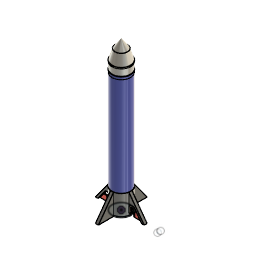
Zephyr I v11 (Autodesk Fusion 360 design; units mm, degrees)
Autodesk Fusion 360 part; units mm, degrees
note: some values were not read from the file. Chosen so that the rebuilt part matches the saved one: which bodies a step acts on; which face or edge a step refers to.
sketch "Szkic1" plane through (0, 0, 0) normal (0, 0, 1) x (1, 0, 0)
  circle A0 centre (0, 0) radius 9
  circle A1 centre (0, 0) radius 37.5
  dimension "d1" = 18
  dimension "d2" = 75
  constraint coincident A0.centre A1.centre
  constraint concentric A0 A1
  measures "d1" diameter of A0
  measures "d2" diameter of A1
extrude "Wyciągnięcie proste1" add sketch "Szkic1" along normal blind 99 makes body 1
sketch "Szkic2" plane through (0, 0, 0) normal (0, 0, 1) x (1, 0, 0)
  circle A0 centre (0, 0) radius 9
  dimension "d5" = 18
  constraint coincident A0.centre origin
  measures "d5" diameter of A0
extrude "Wyciągnięcie proste2" add sketch "Szkic2" along normal blind 30 bodies 1
move_body "Przesuń1" bodies 1 to x (-1, 0, 0) y (0, 1, 0) z (0, 0, -1) at (0, 0, 100)
sketch "Szkic3" plane through (0, 0, 0) normal (0, 1, 0) x (1, 0, 0)
move_face "Odsuń powierzchnie1" offset -20 1 faces at (-8.8919, -13.3334, 100) on bodies 1
sketch "Szkic4" plane through (0, 0, 0) normal (0, 1, 0) x (1, 0, 0)
  line L0 (0, 0) -> (6.25, 0)
  line L1 (0, 0) -> (-6.25, 0)
  line L2 (6.25, 0) -> (6.25, -22.4)
  line L3 (-6.25, 0) -> (-6.25, -22.4)
  line L4 (-6.25, -22.4) -> (6.25, -22.4)
  dimension "d9" = 6.25
  dimension "d10" = 6.25
  dimension "d11" = 22.4
  dimension "d12" = 22.4
  constraint coincident L0.start L1.start
  constraint horizontal L0
  constraint parallel L0 L1
  constraint perpendicular L0 L2
  constraint perpendicular L1 L3
  measures "d9" distance of L0.start L0.end
  measures "d10" distance of L0.start L1.end
  measures "d11" distance of L0.end L2.end
  measures "d12" distance of L1.end L3.end
move_body "Przesuń2" bodies 1 to x (1, 0, 0) y (0, 1, 0) z (0, 0, 1) at (0, 0, -10)
move_body "Przesuń3" bodies 1 to x (1, 0, 0) y (0, 1, 0) z (0, 0, 1) at (0, -40, 0)
move_body "Przesuń4" bodies 1 to x (1, 0, 0) y (0, 1, 0) z (0, 0, 1) at (0, 2.5, 0)
extrude "Wyciągnięcie proste3" cut sketch "Szkic4" against normal blind 19.8 bodies 1
move_body "Przesuń5" bodies 1 to x (1, 0, 0) y (0, 1, 0) z (0, 0, 1) at (0, -2.5, 0)
move_body "Przesuń6" bodies 1 to x (1, 0, 0) y (0, 1, 0) z (0, 0, 1) at (0, 40, 0)
sketch "Szkic6" plane through (0, 0, 0) normal (1, 0, 0) x (0, 1, 0)
  line L0 (0, 0) -> (-6.25, 0)
  line L1 (0, 0) -> (6.25, 0)
  line L2 (6.25, 0) -> (6.25, 22.4)
  line L3 (-6.25, 0) -> (-8, 0)
  line L4 (-8, 0) -> (-8, 22.4)
  line L5 (-8, 22.4) -> (-6.25, 22.4)
  line L6 (-6.25, 22.4) -> (-6.25, 0)
  line L7 (-6.25, 22.4) -> (6.25, 22.4)
  dimension "d22" = 6.25
  dimension "d23" = 6.25
  dimension "d24" = 22.4
  dimension "d25" = 22.4
  constraint coincident L0.start L1.start
  constraint horizontal L0
  constraint parallel L0 L1
  constraint perpendicular L1 L2
  constraint horizontal L3
  constraint vertical L4
  constraint horizontal L5
  constraint vertical L6
  measures "d22" distance of L0.start L0.end
  measures "d23" distance of L0.start L1.end
  measures "d24" distance of L1.end L2.end
  measures "d25" distance of L0.end L5.end
move_body "Przesuń10" bodies 1 to x (0, 1, 0) y (-1, 0, 0) z (0, 0, 1) at (0, 0, 0)
move_body "Przesuń11" bodies 1 to x (1, 0, 0) y (0, 1, 0) z (0, 0, 1) at (-40, 0, 0)
move_body "Przesuń12" bodies 1 to x (1, 0, 0) y (0, 1, 0) z (0, 0, 1) at (2.5, 0, 0)
extrude "Wyciągnięcie proste5" cut sketch "Szkic6" against normal blind 19.8 contours L0 L1 L2 L6 L7 bodies 1
move_body "Przesuń13" bodies 1 to x (1, 0, 0) y (0, 1, 0) z (0, 0, 1) at (2.5, 0, 0)
move_body "Przesuń14" bodies 1 to x (1, 0, 0) y (0, 1, 0) z (0, 0, 1) at (-2.5, 0, 0)
move_body "Przesuń15" bodies 1 to x (1, 0, 0) y (0, 1, 0) z (0, 0, 1) at (-2.5, 0, 0)
move_body "Przesuń16" bodies 1 to x (1, 0, 0) y (0, 1, 0) z (0, 0, 1) at (40, 0, 0)
sketch "Szkic7" plane through (0, 0, 0) normal (1, 0, 0) x (0, 1, 0)
  line L0 (-6.25, 0, 150) -> (6.25, 0, 150)
sketch "Szkic8" plane through (0, 0, 0) normal (0, 0, 1) x (1, 0, 0)
  line L0 (17.7, 6.25) -> (17.7, -6.25)
  line L1 (17.7, -6.25) -> (22.7, -6.25)
  line L2 (22.7, -6.25) -> (22.7, 6.25)
  line L3 (17.7, 6.25) -> (22.7, 6.25)
  line L4 (-17.7, 6.25) -> (-17.7, -6.25)
  line L5 (-17.7, -6.25) -> (-22.7, -6.25)
  line L6 (-22.7, -6.25) -> (-22.7, 6.25)
  line L7 (-22.7, 6.25) -> (-17.7, 6.25)
  dimension "d28" = 12.5
  dimension "d29" = 5
  dimension "d30" = 12.5
  dimension "d31" = 12.5
  dimension "d32" = 5
  dimension "d33" = 12.5
  constraint vertical L0
  constraint perpendicular L0 L1
  constraint perpendicular L1 L2
  constraint vertical L4
  constraint perpendicular L4 L5
  constraint perpendicular L5 L6
  measures "d28" distance of L0.start L0.end
  measures "d29" distance of L0.end L1.end
  measures "d30" distance of L1.end L2.end
  measures "d31" distance of L4.start L4.end
  measures "d32" distance of L4.end L5.end
  measures "d33" distance of L5.end L6.end
extrude "Wyciągnięcie proste6" cut sketch "Szkic8" along normal blind 90 bodies 1
other "Element bazowy siatki1"
other "Element bazowy siatki2"
other "Element bazowy siatki3"
other "Zmień1"
other "Zmień2"
other "Kopiowanie i wklejenie siatek1"
other "Zmień3"
other "Zmień4"
other "Zmień5"
other "Zmień6"
other "Zmień7"
other "Zmień8"
other "Zmień9"
other "Kopiowanie i wklejenie siatek2"
other "Zmień10"
other "Zmień11"
other "Zmień12"
other "Zmień13"
other "Zmień14"
other "Zmień15"
move_body "Przesuń17" bodies 1 to x (1, 0, 0) y (0, 1, 0) z (0, 0, 1) at (0, 0, 10)
other "Zmień16"
sketch "Szkic9" plane through (0, 0, 0) normal (0, 1, 0) x (1, 0, 0)
  line L0 (37.5, -80) -> (95.7821, 0.0262)
  line L1 (-37.5, -80) -> (-95.8898, -0.0523)
  line L2 (-95.8898, -0.0523) -> (-85.8898, -0.0523)
  line L3 (95.7821, 0.0262) -> (85.7821, 0.0262)
  line L4 (37.5, -80) -> (37.5, -37.25)
  line L5 (37.5, -37.25) -> (68.6343, -37.25)
  line L6 (-37.5, -37.2753) -> (-37.5, -80)
  line L7 (-37.5, -37.2753) -> (-68.704, -37.2753)
  line L8 (37.5, -37.25) -> (-37.5, -37.2753)
  line L9 (-37.5, -37.25) -> (-68.7225, -37.25)
  line L10 (85.7821, 0.0262) -> (58.6343, -37.25)
  line L11 (-85.8898, -0.0523) -> (-58.7225, -37.25)
  dimension "d36" = 99
  dimension "d37" = 99
  dimension "d38" = 10
  dimension "d39" = 10
  constraint horizontal L2
  constraint horizontal L3
  constraint vertical L4
  constraint coincident L0 L5.end
  constraint perpendicular L4 L5
  constraint perpendicular L5 L6
  constraint coincident L1 L7.end
  constraint perpendicular L6 L7
  constraint coincident L1 L9.end
  constraint perpendicular L6 L9
  constraint coincident L5 L10.end
  constraint parallel L0 L10
  constraint coincident L9 L11.end
  constraint parallel L1 L11
  measures "d36" distance of L0.start L0.end
  measures "d37" distance of L1.start L1.end
  measures "d38" distance of L1.end L2.end
  measures "d39" distance of L0.end L3.end
move_body "Przesuń18" bodies 1 to x (1, 0, 0) y (0, 1, 0) z (0, 0, 1) at (0, -50, 0)
extrude "Wyciągnięcie proste7" add sketch "Szkic9" along normal blind 6 separate body makes body 2 at (-47.9013, 0, 51.5169) makes body 3 at (-83.5007, 0, 12.4515) makes body 4 at (44.5448, 6, 51.5)
extrude "Wyciągnięcie proste8" add 3 faces at (-83.5007, 0, 12.4515) (-47.9013, 0, 51.5169) (44.5448, 0, 51.5) along direction (0, -1, 0) blind 6 on bodies 2 3 4 bodies 3 2 4
combine "Kombinacja1" operation add target body 2 tool bodies 3 makes body 5 at (-86.834, 2, 12.4515)
move_body "Przesuń19" bodies 1 to x (1, 0, 0) y (0, 1, 0) z (0, 0, 1) at (0, 50, 0)
combine "Kombinacja2" operation add target body 5 tool bodies 2 makes body 6 at (-47.9013, 6, 51.5169)
move_face "Odsuń powierzchnie2" offset 0.028 1 faces at (-58.3027, 2, 37.2753) on bodies 6
combine "Kombinacja3" operation add target body 6 tool bodies 5
copy_body "Kopiuj-wklej bryły2" bodies 4 6 makes body 7 makes body 8
move_body "Przesuń21" bodies 7 8 to x (1, 0, 0) y (0, 1, 0) z (0, 0, 1) at (0, 0, 0)
copy_body "Kopiuj-wklej bryły3" bodies 1 makes body 9
move_body "Przesuń22" bodies 9 to x (1, 0, 0) y (0, 1, 0) z (0, 0, 1) at (0, 0, 0)
sketch "Szkic10" plane through (0, 0, 0) normal (0, 0, 1) x (1, 0, 0)
  circle A0 centre (0, 0) radius 37.5
  dimension "d47" = 75
  constraint coincident A0.centre origin
  measures "d47" diameter of A0
extrude "Wyciągnięcie proste9" add sketch "Szkic10" along normal blind 1 separate body makes body 10
move_body "Przesuń23" bodies 10 7 6 to x (0, -1, 0) y (1, 0, 0) z (0, 0, 1) at (0, 0, 0)
combine "Kombinacja4" operation add target body 10 tool bodies 9
combine "Kombinacja5" operation add target body 1 tool bodies 10
move_face "Odsuń powierzchnie5" offset 37.2 2 faces at (-2, 44.5748, 37.2473) (2, -51.5895, 37.25) on bodies 6 7
sketch "Szkic11" plane through (0, 0, 0) normal (0, 0, 1) x (1, 0, 0)
  circle A0 centre (0, 0) radius 9
  dimension "d51" = 18
  constraint coincident A0.centre origin
  measures "d51" diameter of A0
extrude "Wyciągnięcie proste10" cut sketch "Szkic11" along normal blind 10 bodies 1
sketch "Szkic12" plane through (0, 0, 0) normal (0, 0, 1) x (1, 0, 0)
  circle A0 centre (0, 0) radius 37.5
  dimension "d54" = 75
  constraint coincident A0.centre origin
  measures "d54" diameter of A0
combine "Kombinacja6" operation add target body 4 tool bodies 1
combine "Kombinacja7" operation add target body 4 tool bodies 6
combine "Kombinacja8" operation add target body 4 tool bodies 8
combine "Kombinacja9" operation add target body 7 tool bodies 4
move_body "Przesuń24" bodies 7 to x (1, 0, 0) y (0, 1, 0) z (0, 0, 1) at (0, 0, -80)
other "Zmień17"
sketch "Szkic13" plane through (0, 0, 0) normal (0, 0, 1) x (1, 0, 0)
  circle A0 centre (0, 0) radius 36.5
  dimension "d55" = 73
  constraint coincident A0.centre origin
  measures "d55" diameter of A0
extrude "Wyciągnięcie proste11" add sketch "Szkic12" along normal blind 400 separate body makes body 11
sketch "Szkic14" plane through (0, 0, 0) normal (0, 0, 1) x (1, 0, 0)
  circle A0 centre (0, 0) radius 36.5
  dimension "d58" = 73
  constraint coincident A0.centre origin
  measures "d58" diameter of A0
extrude "Wyciągnięcie proste12" cut sketch "Szkic13" along normal blind 500 bodies 11
sketch "Szkic15" plane through (0, 0, 0) normal (0, 0, 1) x (1, 0, 0)
  circle A0 centre (0, 0) radius 10
  circle A1 centre (0, 0) radius 9
  dimension "d61" = 20
  dimension "d62" = 18
  constraint coincident A0.centre A1.centre
  constraint concentric A0 A1
  measures "d61" diameter of A0
  measures "d62" diameter of A1
extrude "Wyciągnięcie proste13" cut sketch "Szkic15" against normal blind 130 bodies 7 makes body 12 at (6, -53.5755, -53.3) makes body 12 at (-36.0833, 10.2102, -42.5333) makes body 12 at (-76.4265, 0.0026, -53.2985) makes body 12 at (-6, 56.9645, -53.3018) makes body 12 at (76.3547, -0.0026, -53.3508)
sketch "Szkic16" plane through (0, 0, 0) normal (0, 0, 1) x (1, 0, 0)
  circle A0 centre (0, 0) radius 10
  circle A1 centre (0, 0) radius 9
  dimension "d65" = 20
  dimension "d66" = 18
  constraint coincident A0.centre A1.centre
  constraint concentric A0 A1
  measures "d65" diameter of A0
  measures "d66" diameter of A1
move_body "Przesuń25" bodies 12 11 to x (1, 0, 0) y (0, 1, 0) z (0, 0, 1) at (0, -120, 0)
other "Zmień18"
extrude "Wyciągnięcie proste14" add sketch "Szkic16" against normal blind 80 bodies 7
move_body "Przesuń26" bodies 11 12 to x (1, 0, 0) y (0, 1, 0) z (0, 0, 1) at (0, 120, 0)
other "Zmień19"
move_body "Przesuń27" bodies 11 12 to x (1, 0, 0) y (0, 1, 0) z (0, 0, 1) at (0, 0, 80)
other "Zmień20"
move_body "Przesuń28" bodies 7 to x (1, 0, 0) y (0, 1, 0) z (0, 0, 1) at (0, 0, 80)
sketch "Szkic17" plane through (0, 0, 0) normal (0, 1, 0) x (1, 0, 0)
  line L0 (54.3, 0.55) -> (54.3, -36.5257)
  line L1 (54.3, -36.5257) -> (58.3, -36.5257)
  line L2 (58.3, -36.5257) -> (85, 0)
  line L3 (85, 0) -> (54.3, 0.55)
  line L4 (-53.9, 0.55) -> (-54.1253, -36.5257)
  line L5 (-54.1253, -36.5257) -> (-58.1253, -36.5014)
  line L6 (-58.1253, -36.5014) -> (-85, 0)
  line L7 (-85, 0) -> (-53.9, 0.55)
  line L8 (-54.0249, -19.9942) -> (-70.2789, -19.9942)
  line L9 (54.3, -19.9942) -> (70.3844, -19.9942)
  dimension "d69" = 4
  dimension "d70" = 4
  constraint vertical L0
  constraint perpendicular L0 L1
  constraint perpendicular L4 L5
  constraint coincident L4 L8.start
  constraint coincident L6 L8.end
  constraint horizontal L8
  constraint coincident L0 L9.start
  constraint coincident L2 L9.end
  constraint perpendicular L0 L9
  measures "d69" distance of L0.end L1.end
  measures "d70" distance of L4.end L5.end
extrude "Wyciągnięcie proste15" add sketch "Szkic17" along normal blind 2 separate body contours L0 L2 L3 L9 | L4 L6 L7 L8 makes body 13 at (-69.7263, 0, 6.4814) makes body 14 at (69.8948, 0, 6.4814)
move_face "Odsuń powierzchnie6" offset 2 2 faces at (-69.7263, 0, 6.4814) (69.8948, 0, 6.4814) on bodies 13 14
move_body "Przesuń29" bodies 14 11 12 13 7 to x (1, 0, 0) y (0, 1, 0) z (0, 0, 1) at (0, 0, -480)
other "Zmień21"
move_body "Przesuń30" bodies 7 14 13 12 11 to x (1, 0, 0) y (0, 1, 0) z (0, 0, 1) at (0, 0, -25)
other "Zmień22"
sketch "Szkic19" plane through (0, 0, 0) normal (0, 0, 1) x (1, 0, 0)
  circle A0 centre (0, 0) radius 36.5
  circle A1 centre (0, 0) radius 37.5
  circle A2 centre (0, 0) radius 35.5
  dimension "d75" = 73
  dimension "d76" = 75
  dimension "d77" = 71
  constraint coincident A0.centre A1.centre
  constraint concentric A0 A2
  measures "d75" diameter of A0
  measures "d76" diameter of A1
  measures "d77" diameter of A2
extrude "Wyciągnięcie proste16" add sketch "Szkic19" against normal blind 10 separate body contours A0 makes body 15
sketch "Szkic20" plane through (0, 0, 0) normal (0, 0, 1) x (1, 0, 0)
  circle A0 centre (0, 0) radius 37.5
  dimension "d80" = 75
  constraint coincident A0.centre origin
  measures "d80" diameter of A0
extrude "Wyciągnięcie proste17" add sketch "Szkic20" along normal blind 2 bodies 15
move_body "Przesuń31" bodies 15 to x (1, 0, 0) y (0, 1, 0) z (0, 0, 1) at (0, 0, -2)
sketch "Szkic21" plane through (0, 0, 0) normal (0, 0, 1) x (1, 0, 0)
  circle A0 centre (0, 0) radius 37.5
  circle A1 centre (0, 0) radius 36.5
  dimension "d83" = 75
  dimension "d84" = 73
  constraint coincident A0.centre A1.centre
  measures "d83" diameter of A0
  measures "d84" diameter of A1
extrude "Wyciągnięcie proste18" add sketch "Szkic21" along normal blind 30 bodies 15
move_body "Przesuń32" bodies 15 11 12 14 13 to x (1, 0, 0) y (0, 1, 0) z (0, 0, 1) at (0, 0, -40)
other "Zmień23"
sketch "Szkic22" plane through (0, 0, 0) normal (0, 1, 0) x (1, 0, 0)
  line L0 (0, 0) -> (37.5, 0)
  line L1 (0, 0) -> (0, -75)
  line L2 (37.5, 0) -> (25, -40)
  line L3 (25, -40) -> (0, -75)
  dimension "d87" = 37.5
  dimension "d88" = 75
  constraint coincident L0.start L1.start
  constraint horizontal L0
  constraint perpendicular L0 L1
  measures "d87" distance of L0.start L0.end
  measures "d88" distance of L0.start L1.end
revolve "Obrót1" add sketch "Szkic22" angle 360 about axis through (0, 0, 0) along (0, 0, 1) separate body makes body 16
sketch "Szkic23" plane through (0, 0, 0) normal (0, 0, 1) x (1, 0, 0)
  circle A0 centre (0, 0) radius 36.5
  dimension "d90" = 73
  constraint coincident A0.centre origin
  measures "d90" diameter of A0
sketch "Szkic24" plane through (0, 0, 0) normal (0, 0, 1) x (1, 0, 0)
  circle A0 centre (0, 0) radius 35.5
  dimension "d91" = 71
  constraint coincident A0.centre origin
  measures "d91" diameter of A0
extrude "Wyciągnięcie proste19" add sketch "Szkic14" against normal blind 5 bodies 16
move_body "Przesuń33" bodies 16 to x (1, 0, 0) y (0, 1, 0) z (0, 0, 1) at (0, 0, 50)
sketch "Szkic25" plane through (0, 0, 0) normal (0, 0, 1) x (1, 0, 0)
  circle A0 centre (0, 0) radius 35.5
  dimension "d94" = 71
  constraint coincident A0.centre origin
  measures "d94" diameter of A0
extrude "Wyciągnięcie proste20" cut sketch "Szkic25" along normal blind 50 bodies 16
move_body "Przesuń34" bodies 13 12 14 15 16 to x (1, 0, 0) y (0, 1, 0) z (0, 0, 1) at (0, 0, 545)
other "Zmień24"
move_body "Przesuń35" bodies 11 to x (1, 0, 0) y (0, 1, 0) z (0, 0, 1) at (0, 0, 550)
move_body "Przesuń36" bodies 7 to x (1, 0, 0) y (0, 1, 0) z (0, 0, 1) at (0, 0, 505)
move_body "Przesuń37" bodies 11 to x (1, 0, 0) y (0, 1, 0) z (0, 0, 1) at (0, 0, -5)
move_body "Przesuń38" bodies 15 to x (1, 0, 0) y (0, 1, 0) z (0, 0, 1) at (0, 0, -23)
move_body "Przesuń39" bodies 16 to x (1, 0, 0) y (0, 1, 0) z (0, 0, 1) at (0, 0, -83)
split "Podział1" by face at (-36.0833, 10.2102, 37.4667) of body 12 bodies 12 makes body 17 at (76.3547, -0.0026, 26.6492) makes body 18 at (-76.4265, 0.0026, 26.7015) makes body 19 at (-6, 56.9645, 26.6982) makes body 20 at (6, -53.5755, 26.7)
move_body "Przesuń40" bodies 19 to x (1, 0, 0) y (0, 1, 0) z (0, 0, 1) at (0, -1, 0)
move_face "Odsuń powierzchnie7" offset -2 1 faces at (75.2563, 0.6667, 13.3295) on bodies 14
move_face "Odsuń powierzchnie8" offset -2 1 faces at (-75.186, -0.6667, 13.3295) on bodies 13
move_body "Przesuń41" bodies 18 to x (1, 0, 0) y (0, 1, 0) z (0, 0, 1) at (1, 0, 0)
move_body "Przesuń42" bodies 17 to x (1, 0, 0) y (0, 1, 0) z (0, 0, 1) at (-1, 0, 0)
move_body "Przesuń43" bodies 20 to x (1, 0, 0) y (0, 1, 0) z (0, 0, 1) at (0, 1, 0)
move_face "Odsuń powierzchnie9" offset -0.5 1 faces at (-24.2805, 0.6973, 10) on bodies 12
move_face "Odsuń powierzchnie10" offset -0.5 1 faces at (24.2805, 0.6973, 10) on bodies 12
move_face "Odsuń powierzchnie11" offset -0.5 1 faces at (24.2805, 0.6973, 9.5) on bodies 12
move_face "Odsuń powierzchnie12" offset -0.5 1 faces at (-24.2805, 0.6973, 9.5) on bodies 12
move_body "Przesuń44" bodies 19 to x (1, 0, 0) y (0, 1, 0) z (0, 0, 1) at (0, -1, 0)
move_body "Przesuń45" bodies 20 to x (1, 0, 0) y (0, 1, 0) z (0, 0, 1) at (0, 1, 0)
move_body "Przesuń46" bodies 18 to x (1, 0, 0) y (0, 1, 0) z (0, 0, 1) at (1, 0, 0)
move_body "Przesuń47" bodies 17 to x (1, 0, 0) y (0, 1, 0) z (0, 0, 1) at (-1, 0, 0)
sketch "Szkic26" plane through (0, 0, 0) normal (0, 0, 1) x (1, 0, 0)
  circle A0 centre (0, 0) radius 12.5
  circle A1 centre (0, 0) radius 7.5
  line L0 (11, -5) -> (22.5, -5)
  line L1 (22.5, -5) -> (22.5, 5)
  line L2 (22.5, 5) -> (11, 5)
  line L3 (-11, 5) -> (-22.5, 5)
  line L4 (-22.5, -5) -> (-22.5, 5)
  line L5 (-22.5, -5) -> (-11, -5)
  dimension "d103" = 25
  dimension "d104" = 15
  constraint coincident A0.centre A1.centre
  constraint concentric A0 A1
  constraint horizontal L0
  constraint perpendicular L0 L1
  constraint perpendicular L1 L2
  constraint horizontal L3
  constraint perpendicular L3 L4
  constraint perpendicular L4 L5
  measures "d103" diameter of A0
  measures "d104" diameter of A1
move_body "Przesuń48" bodies 12 to x (1, 0, 0) y (0, 1, 0) z (0, 0, 1) at (0, 0, -120)
move_body "Przesuń49" bodies 7 to x (1, 0, 0) y (0, 1, 0) z (0, 0, 1) at (0, 0, 3)
extrude "Wyciągnięcie proste21" add sketch "Szkic26" against normal blind 3 separate body makes body 21
move_body "Przesuń50" bodies 7 to x (1, 0, 0) y (0, 1, 0) z (0, 0, 1) at (0, 0, -3)
move_body "Przesuń51" bodies 12 to x (1, 0, 0) y (0, 1, 0) z (0, 0, 1) at (0, 0, 120)
move_face "Odsuń powierzchnie13" offset 4 5 faces at (-90.5565, 2, 0.0523) (0.0026, 74.429, 0.0473) (90.4487, 2, -0.0262) (2, -87.1154, -0.0262) (0, -67.651, 0.05) on bodies 17 18 19 20
sketch "Szkic27" plane through (0, 0, 0) normal (0, 0, 1) x (1, 0, 0)
sketch "Szkic28" plane through (0, 0, 0) normal (0, 0, 1) x (1, 0, 0)
  circle A0 centre (17.5, 0) radius 1.5
  circle A1 centre (-17.5, 0) radius 1.5
  dimension "d108" = 3
  dimension "d109" = 3
  measures "d108" diameter of A0
  measures "d109" diameter of A1
move_body "Przesuń52" bodies 11 17 12 19 18 13 21 15 16 20 14 7 to x (1, 0, 0) y (0, 1, 0) z (0, 0, 1) at (0, 0, 3)
other "Zmień25"
extrude "Wyciągnięcie proste22" cut sketch "Szkic28" along normal blind 6 bodies 12 21
